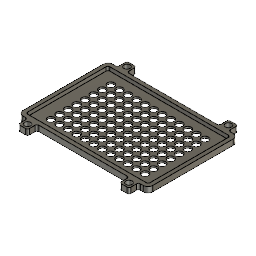
Assembled (Autodesk Fusion 360 archive; units mm, degrees)
design "Plate_Adapter_96"
Autodesk Fusion 360 part; units mm, degrees
note: some values were not read from the file. Chosen so that the rebuilt part matches the saved one: which face or edge a step refers to; which pieces of a blend or face edit are solid. Set by a fixed rule: which sketch regions a step uses.
sketch "Sketch1" plane through (0, 0, 0) normal (0, 0, 1) x (1, 0, 0)
  line L0 (-68.38, 47.37) -> (68.38, 47.37)
  line L1 (68.38, 47.37) -> (68.38, -47.37)
  line L2 (68.38, -47.37) -> (-68.38, -47.37)
  line L3 (-68.38, -47.37) -> (-68.38, 47.37)
  line L4 (-68.38, 47.37) -> (68.38, -47.37) construction
  line L5 (68.38, 47.37) -> (-68.38, -47.37) construction
  line L6 (-58.38, 57.37) -> (-48.38, 57.37)
  line L7 (-48.38, 57.37) -> (-48.38, 47.37)
  line L8 (-48.38, 47.37) -> (-58.38, 47.37)
  line L9 (-58.38, 47.37) -> (-58.38, 57.37)
  line L10 (48.38, 57.37) -> (58.38, 57.37)
  line L11 (58.38, 57.37) -> (58.38, 47.37)
  line L12 (58.38, 47.37) -> (48.38, 47.37)
  line L13 (48.38, 47.37) -> (48.38, 57.37)
  line L14 (48.38, -47.37) -> (58.38, -47.37)
  line L15 (58.38, -47.37) -> (58.38, -57.37)
  line L16 (58.38, -57.37) -> (48.38, -57.37)
  line L17 (48.38, -57.37) -> (48.38, -47.37)
  line L18 (-58.38, -47.37) -> (-48.38, -47.37)
  line L19 (-48.38, -47.37) -> (-48.38, -57.37)
  line L20 (-48.38, -57.37) -> (-58.38, -57.37)
  line L21 (-58.38, -57.37) -> (-58.38, -47.37)
  line L22 (-49.5, 31.5) -> (49.5, 31.5)
  line L23 (49.5, 31.5) -> (49.5, -31.5)
  line L24 (49.5, -31.5) -> (-49.5, -31.5)
  line L25 (-49.5, -31.5) -> (-49.5, 31.5)
  line L26 (-49.5, 31.5) -> (49.5, -31.5) construction
  line L27 (49.5, 31.5) -> (-49.5, -31.5) construction
  circle A0 centre (-49.5, -31.5) radius 3.575
  circle A1 centre (-40.5, -31.5) radius 3.575
  circle A2 centre (-31.5, -31.5) radius 3.575
  circle A3 centre (-22.5, -31.5) radius 3.575
  circle A4 centre (-13.5, -31.5) radius 3.575
  circle A5 centre (-4.5, -31.5) radius 3.575
  circle A6 centre (4.5, -31.5) radius 3.575
  circle A7 centre (13.5, -31.5) radius 3.575
  circle A8 centre (22.5, -31.5) radius 3.575
  circle A9 centre (31.5, -31.5) radius 3.575
  circle A10 centre (40.5, -31.5) radius 3.575
  circle A11 centre (49.5, -31.5) radius 3.575
  circle A12 centre (-49.5, -22.5) radius 3.575
  circle A13 centre (-40.5, -22.5) radius 3.575
  circle A14 centre (-31.5, -22.5) radius 3.575
  circle A15 centre (-22.5, -22.5) radius 3.575
  circle A16 centre (-13.5, -22.5) radius 3.575
  circle A17 centre (-4.5, -22.5) radius 3.575
  circle A18 centre (4.5, -22.5) radius 3.575
  circle A19 centre (13.5, -22.5) radius 3.575
  circle A20 centre (22.5, -22.5) radius 3.575
  circle A21 centre (31.5, -22.5) radius 3.575
  circle A22 centre (40.5, -22.5) radius 3.575
  circle A23 centre (49.5, -22.5) radius 3.575
  circle A24 centre (-49.5, -13.5) radius 3.575
  circle A25 centre (-40.5, -13.5) radius 3.575
  circle A26 centre (-31.5, -13.5) radius 3.575
  circle A27 centre (-22.5, -13.5) radius 3.575
  circle A28 centre (-13.5, -13.5) radius 3.575
  circle A29 centre (-4.5, -13.5) radius 3.575
  circle A30 centre (4.5, -13.5) radius 3.575
  circle A31 centre (13.5, -13.5) radius 3.575
  circle A32 centre (22.5, -13.5) radius 3.575
  circle A33 centre (31.5, -13.5) radius 3.575
  circle A34 centre (40.5, -13.5) radius 3.575
  circle A35 centre (49.5, -13.5) radius 3.575
  circle A36 centre (-49.5, -4.5) radius 3.575
  circle A37 centre (-40.5, -4.5) radius 3.575
  circle A38 centre (-31.5, -4.5) radius 3.575
  circle A39 centre (-22.5, -4.5) radius 3.575
  circle A40 centre (-13.5, -4.5) radius 3.575
  circle A41 centre (-4.5, -4.5) radius 3.575
  circle A42 centre (4.5, -4.5) radius 3.575
  circle A43 centre (13.5, -4.5) radius 3.575
  circle A44 centre (22.5, -4.5) radius 3.575
  circle A45 centre (31.5, -4.5) radius 3.575
  circle A46 centre (40.5, -4.5) radius 3.575
  circle A47 centre (49.5, -4.5) radius 3.575
  circle A48 centre (-49.5, 4.5) radius 3.575
  circle A49 centre (-40.5, 4.5) radius 3.575
  circle A50 centre (-31.5, 4.5) radius 3.575
  circle A51 centre (-22.5, 4.5) radius 3.575
  circle A52 centre (-13.5, 4.5) radius 3.575
  circle A53 centre (-4.5, 4.5) radius 3.575
  circle A54 centre (4.5, 4.5) radius 3.575
  circle A55 centre (13.5, 4.5) radius 3.575
  circle A56 centre (22.5, 4.5) radius 3.575
  circle A57 centre (31.5, 4.5) radius 3.575
  circle A58 centre (40.5, 4.5) radius 3.575
  circle A59 centre (49.5, 4.5) radius 3.575
  circle A60 centre (-49.5, 13.5) radius 3.575
  circle A61 centre (-40.5, 13.5) radius 3.575
  circle A62 centre (-31.5, 13.5) radius 3.575
  circle A63 centre (-22.5, 13.5) radius 3.575
  circle A64 centre (-13.5, 13.5) radius 3.575
  circle A65 centre (-4.5, 13.5) radius 3.575
  circle A66 centre (4.5, 13.5) radius 3.575
  circle A67 centre (13.5, 13.5) radius 3.575
  circle A68 centre (22.5, 13.5) radius 3.575
  circle A69 centre (31.5, 13.5) radius 3.575
  circle A70 centre (40.5, 13.5) radius 3.575
  circle A71 centre (49.5, 13.5) radius 3.575
  circle A72 centre (-49.5, 22.5) radius 3.575
  circle A73 centre (-40.5, 22.5) radius 3.575
  circle A74 centre (-31.5, 22.5) radius 3.575
  circle A75 centre (-22.5, 22.5) radius 3.575
  circle A76 centre (-13.5, 22.5) radius 3.575
  circle A77 centre (-4.5, 22.5) radius 3.575
  circle A78 centre (4.5, 22.5) radius 3.575
  circle A79 centre (13.5, 22.5) radius 3.575
  circle A80 centre (22.5, 22.5) radius 3.575
  circle A81 centre (31.5, 22.5) radius 3.575
  circle A82 centre (40.5, 22.5) radius 3.575
  circle A83 centre (49.5, 22.5) radius 3.575
  circle A84 centre (-49.5, 31.5) radius 3.575
  circle A85 centre (-40.5, 31.5) radius 3.575
  circle A86 centre (-31.5, 31.5) radius 3.575
  circle A87 centre (-22.5, 31.5) radius 3.575
  circle A88 centre (-13.5, 31.5) radius 3.575
  circle A89 centre (-4.5, 31.5) radius 3.575
  circle A90 centre (4.5, 31.5) radius 3.575
  circle A91 centre (13.5, 31.5) radius 3.575
  circle A92 centre (22.5, 31.5) radius 3.575
  circle A93 centre (31.5, 31.5) radius 3.575
  circle A94 centre (40.5, 31.5) radius 3.575
  circle A95 centre (49.5, 31.5) radius 3.575
  point P0 (-57.3369, -42.2056)
  point P1 (-53.88, -84.89)
  dimension "d1" = 136.76
  dimension "d2" = 94.74
  dimension "d3" = 10
  dimension "d4" = 10
  dimension "d5" = 10
  dimension "d6" = 10
  dimension "d7" = 63
  dimension "d8" = 99
  dimension "d10" = 7.15
  dimension "d13" = 99
  dimension "d14" = 63
  constraint perpendicular L0 L1
  constraint parallel L0 L2
  constraint parallel L1 L3
  constraint horizontal L0
  constraint coincident L4 origin
  constraint coincident L5 origin
  constraint horizontal L6
  constraint vertical L7
  constraint horizontal L8
  constraint vertical L9
  constraint coincident L0 L7.end
  constraint horizontal L10
  constraint vertical L11
  constraint horizontal L12
  constraint vertical L13
  constraint horizontal L14
  constraint vertical L15
  constraint horizontal L16
  constraint vertical L17
  constraint horizontal L18
  constraint vertical L19
  constraint horizontal L20
  constraint vertical L21
  constraint perpendicular L22 L23
  constraint parallel L22 L24
  constraint parallel L23 L25
  constraint horizontal L22
  constraint coincident L26 origin
  constraint coincident L27 origin
  measures "d1" distance of L1 L3
  measures "d2" distance of L0.start L2.end
  measures "d3" distance of L6.start L6.end
  measures "d4" distance of L6.start L8.end
  measures "d5" distance of L10.start L10.end
  measures "d6" distance of L10.start L12.end
  measures "d7" distance of L22.end L23.end
  measures "d8" distance of L23.end L24.end
  measures "d10" diameter of A0
extrude "Extrude1" add sketch "Sketch1" along normal mid plane 6 contours L0 L1 L2 L3 L8 L12 L14 L18 | L0 L6 L7 L8 L9 | L2 L18 L19 L20 L21 | L0 L10 L11 L12 L13 | L2 L14 L15 L16 L17 | L22 L23 L24 L25 A0 A1 A2 A3 A4 A5 A6 A7 A8 A9 A10 A11 A12 A23 A24 A35 A36 A47 A48 A59 A60 A71 A72 A83 A84 A85 A86 A87 A88 A89 A90 A91 A92 A93 A94 A95
ref_plane "WorkPlane1" through (0, 0, 3) normal (0, 0, 1) x (1, 0, 0)
sketch "Sketch2" plane through (0, 0, 3) normal (0, 0, 1) x (1, 0, 0)
  line L0 (-64.38, 43.235) -> (64.38, 43.235)
  line L1 (64.38, 43.235) -> (64.38, -43.235)
  line L2 (64.38, -43.235) -> (-64.38, -43.235)
  line L3 (-64.38, -43.235) -> (-64.38, 43.235)
  line L4 (-64.38, 43.235) -> (64.38, -43.235) construction
  line L5 (64.38, 43.235) -> (-64.38, -43.235) construction
  dimension "d18" = 128.76
  dimension "d19" = 86.47
  constraint perpendicular L0 L1
  constraint parallel L0 L2
  constraint parallel L1 L3
  constraint horizontal L0
  constraint coincident L4 origin
  constraint coincident L5 origin
  measures "d18" distance of L1.end L2.end
  measures "d19" distance of L0.end L1.end
extrude "Extrude2" cut sketch "Sketch2" against normal blind 4
sketch "Sketch3" plane through (0, 0, 3) normal (0, 0, 1) x (-1, 0, 0)
  line L0 (-64.38, -43.235) -> (-64.38, 43.235)
  line L1 (-64.38, 43.235) -> (64.38, 43.235)
  line L2 (64.38, 43.235) -> (64.38, -43.235)
  line L3 (64.38, -43.235) -> (-64.38, -43.235)
  line L4 (58.38, 57.37) -> (48.38, 57.37)
  line L5 (48.38, 57.37) -> (48.38, 47.37)
  line L6 (48.38, 47.37) -> (-48.38, 47.37)
  line L7 (-48.38, 47.37) -> (-48.38, 57.37)
  line L8 (-48.38, 57.37) -> (-58.38, 57.37)
  line L9 (-58.38, 57.37) -> (-58.38, 47.37)
  line L10 (-58.38, 47.37) -> (-68.38, 47.37)
  line L11 (-68.38, 47.37) -> (-68.38, -47.37)
  line L12 (-68.38, -47.37) -> (-58.38, -47.37)
  line L13 (-58.38, -47.37) -> (-58.38, -57.37)
  line L14 (-58.38, -57.37) -> (-48.38, -57.37)
  line L15 (-48.38, -57.37) -> (-48.38, -47.37)
  line L16 (-48.38, -47.37) -> (48.38, -47.37)
  line L17 (48.38, -47.37) -> (48.38, -57.37)
  line L18 (48.38, -57.37) -> (58.38, -57.37)
  line L19 (58.38, -57.37) -> (58.38, -47.37)
  line L20 (58.38, -47.37) -> (68.38, -47.37)
  line L21 (68.38, -47.37) -> (68.38, 47.37)
  line L22 (68.38, 47.37) -> (58.38, 47.37)
  line L23 (58.38, 47.37) -> (58.38, 57.37)
  circle A0 centre (53.38, -52.37) radius 3.25
  circle A1 centre (-53.38, -52.3704) radius 3.25
  circle A2 centre (-53.38, 52.3703) radius 3.25
  circle A3 centre (53.38, 52.37) radius 3.25
  dimension "d22" = 6.5
  dimension "d23" = 6.5
  dimension "d24" = 6.5
  dimension "d25" = 6.5
  measures "d22" diameter of A0
  measures "d23" diameter of A1
  measures "d24" diameter of A2
  measures "d25" diameter of A3
extrude "Extrude3" cut sketch "Sketch3" against normal blind 6 contours A0 | A1 | A2 | A3
fillet "Fillet1" radius 5 4 edges at (68.38, -47.37, 0) (68.38, 47.37, 0) (-68.38, -47.37, 0) (-68.38, 47.37, 0)
fillet "Fillet2" radius 2 4 edges at (64.38, 43.235, 1) (-64.38, 43.235, 1) (-64.38, -43.235, 1) (64.38, -43.235, 1)
fillet "Fillet3" radius 2 16 edges at (48.38, 47.37, 0) (48.38, 57.37, 0) (58.38, 57.37, 0) (-58.38, 47.37, 0) (-58.38, 57.37, 0) (-48.38, 57.37, 0) (-48.38, 47.37, 0) (58.38, 47.37, 0) (58.38, -47.37, 0) (58.38, -57.37, 0) (48.38, -57.37, 0) (-48.38, -47.37, 0) (-48.38, -57.37, 0) (48.38, -47.37, 0) (-58.38, -47.37, 0) (-58.38, -57.37, 0)

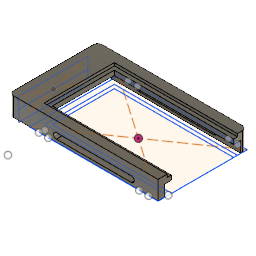
design "Mounting_plate_96_v3 (no bolt holes)"
Autodesk Fusion 360 part; units mm, degrees
sketch "Sketch1" plane through (0, 0, 0) normal (0, 0, 1) x (1, 0, 0)
  line L0 (-68.38, 47.37) -> (68.38, 47.37)
  line L1 (68.38, 47.37) -> (68.38, -47.37)
  line L2 (68.38, -47.37) -> (-68.38, -47.37)
  line L3 (-68.38, -47.37) -> (-68.38, 47.37)
  line L4 (-68.38, 47.37) -> (68.38, -47.37) construction
  line L5 (68.38, 47.37) -> (-68.38, -47.37) construction
  line L6 (-48.38, 47.37) -> (-58.38, 47.37)
  line L7 (58.38, 47.37) -> (48.38, 47.37)
  line L8 (48.38, -47.37) -> (58.38, -47.37)
  line L9 (-58.38, -47.37) -> (-48.38, -47.37)
  line L10 (68.38, 47.37) -> (68.38, 37)
  line L11 (68.38, -47.37) -> (68.38, -36.63)
  line L12 (68.38, 37) -> (-62.58, 37)
  line L13 (-62.58, 37) -> (-62.58, -37)
  line L14 (-62.58, -37) -> (68.38, -37)
  line L15 (68.38, -37) -> (68.38, 37)
  line L16 (68.38, 37) -> (68.38, 33)
  line L17 (68.38, 33) -> (-58.58, 33)
  line L18 (-58.58, 33) -> (-58.58, -33)
  line L19 (-58.58, -33) -> (68.38, -33)
  line L20 (68.38, -33) -> (68.38, 33)
  point P0 (-57.3369, -42.2056)
  point P1 (-53.88, -84.89)
  dimension "d1" = 136.76
  dimension "d2" = 94.74
  dimension "d15" = 10.37
  dimension "d16" = 10.74
  dimension "d17" = 74
  dimension "d18" = 130.96
  dimension "d19" = 4
  dimension "d20" = 66
  dimension "d21" = 126.96
  constraint perpendicular L0 L1
  constraint parallel L0 L2
  constraint parallel L1 L3
  constraint horizontal L0
  constraint horizontal L6
  constraint coincident L0 L6.start
  constraint horizontal L7
  constraint horizontal L8
  constraint horizontal L9
  constraint perpendicular L0 L10
  constraint perpendicular L2 L11
  constraint horizontal L12
  constraint vertical L13
  constraint horizontal L14
  constraint vertical L15
  constraint perpendicular L12 L16
  constraint horizontal L17
  constraint vertical L18
  constraint horizontal L19
  constraint vertical L20
  measures "d1" distance of L1 L3
  measures "d2" distance of L0.start L2.end
  measures "d15" distance of L0.end L10.end
  measures "d16" distance of L1.end L11.end
  measures "d17" distance of L10.end L14.end
  measures "d18" distance of L10.end L12.end
  measures "d19" distance of L10.end L16.end
  measures "d20" distance of L16.end L19.end
  measures "d21" distance of L16.end L17.end
  measures "d160" distance of L0.end
extrude "Extrude2" add sketch "Sketch1" along normal blind 20 contours L0 L1 L2 L3 L6 L7 L8 L9 L10 L11 L12 L13 L14 | L1 L11 L12 L13 L14 L15 L16 L17 L18 L19
ref_plane "WorkPlane2" through (0, 0, 20) normal (0, 0, 1) x (1, 0, 0)
sketch "Sketch4" plane through (0, 0, 20) normal (0, 0, 1) x (1, 0, 0)
  line L0 (68.38, 37) -> (-62.58, 37)
  line L1 (-62.58, 37) -> (-62.58, -37.7)
  line L2 (-62.58, -37.7) -> (68.38, -37.7)
  line L3 (68.38, -37.7) -> (68.38, 37)
  dimension "d30" = 130.96
  dimension "d31" = 74.7
  constraint horizontal L0
  constraint vertical L1
  constraint horizontal L2
  constraint vertical L3
  measures "d30" distance of L0.start L0.end
  measures "d31" distance of L0.start L2.end
extrude "Extrude3" cut sketch "Sketch4" against normal blind 3
ref_plane "WorkPlane3" through (0, 0, 20) normal (0, 0, 1) x (1, 0, 0)
sketch "Sketch5" plane through (0, 0, 20) normal (0, 0, 1) x (1, 0, 0)
  circle A0 centre (-53.38, 52.37) radius 3.25
  circle A1 centre (53.38, 52.37) radius 3.25
  circle A2 centre (-53.38, -52.37) radius 3.25
  circle A3 centre (53.38, -52.37) radius 3.25
  dimension "d35" = 6.5
  dimension "d38" = 106.76
  dimension "d39" = -104.74
  measures "d35" diameter of A0
extrude "Extrude4" cut sketch "Sketch5" against normal blind 20
ref_plane "WorkPlane5" through (68.38, 0, 0) normal (1, 0, 0) x (0, 1, 0)
ref_plane "WorkPlane6" through (68.38, 0, 0) normal (1, 0, 0) x (0, 1, 0)
sketch "Sketch7" plane through (68.38, 0, 0) normal (1, 0, 0) x (0, 1, 0)
  line L0 (40.5, 12) -> (-40.5, 12)
  line L1 (-40.5, 12) -> (-40.5, -12)
  line L2 (-40.5, -12) -> (40.5, -12)
  line L3 (40.5, -12) -> (40.5, 12)
  line L4 (40.5, 12) -> (-40.5, -12) construction
  line L5 (-40.5, 12) -> (40.5, -12) construction
  dimension "d45" = 81
  dimension "d46" = 24
  constraint perpendicular L0 L1
  constraint parallel L0 L2
  constraint parallel L1 L3
  constraint horizontal L0
  constraint coincident L4 origin
  constraint coincident L5 origin
  measures "d45" distance of L1.end L2.end
  measures "d46" distance of L0.end L1.end
extrude "Extrude5" cut sketch "Sketch7" against normal blind 136.76
fillet "Fillet2" [no effect]
ref_plane "WorkPlane7" through (0, -47.37, 10) normal (0, -1, 0) x (1, 0, 0)
delete_face "DeleteFace1" [no effect]
ref_plane "WorkPlane9" through (0, -47.37, 10) normal (0, -1, 0) x (1, 0, 0)
sketch "Sketch10" plane through (0, -47.37, 10) normal (0, -1, 0) x (1, 0, 0)
  line L0 (0, -10) -> (0, -4)
  line L1 (40, -7) -> (-40, -7)
  line L2 (-40, -7) -> (-40, -1)
  line L3 (-40, -1) -> (40, -1)
  line L4 (40, -1) -> (40, -7)
  line L5 (40, -7) -> (-40, -1) construction
  line L6 (-40, -7) -> (40, -1) construction
  circle A0 centre (-40, -4) radius 3
  circle A1 centre (40, -4) radius 3
  point P0 (0, -4)
  dimension "d72" = 6
  dimension "d73" = 6
  dimension "d74" = 80
  dimension "d75" = 6
  dimension "d76" = 6
  constraint vertical L0
  constraint perpendicular L1 L2
  constraint parallel L1 L3
  constraint parallel L2 L4
  constraint horizontal L1
  constraint coincident L5 P0
  constraint coincident L6 P0
  constraint coincident P0 L0.end
  constraint midpoint L2 A0.centre
  constraint midpoint L4 A1.centre
  measures "d72" distance of L0.start P0
  measures "d73" distance of L1.end L2.end
  measures "d74" distance of L2.end L3.end
  measures "d75" diameter of A0
  measures "d76" diameter of A1
extrude "Extrude9" cut sketch "Sketch10" against normal blind 6.87
ref_plane "WorkPlane10" through (0, 47.37, 10) normal (0, 1, 0) x (-1, 0, 0)
sketch "Sketch11" plane through (0, 47.37, 10) normal (0, 1, 0) x (1, 0, 0)
  line L0 (0, 10) -> (0, 4)
  line L1 (-40, 7) -> (40, 7)
  line L2 (40, 7) -> (40, 1)
  line L3 (40, 1) -> (-40, 1)
  line L4 (-40, 1) -> (-40, 7)
  line L5 (-40, 7) -> (40, 1) construction
  line L6 (40, 7) -> (-40, 1) construction
  circle A0 centre (40, 4) radius 3
  circle A1 centre (-40, 4) radius 3
  point P0 (0, 4)
  dimension "d80" = 6
  dimension "d81" = 80
  dimension "d82" = 6
  dimension "d83" = 6
  dimension "d84" = 6
  constraint vertical L0
  constraint perpendicular L1 L2
  constraint parallel L1 L3
  constraint parallel L2 L4
  constraint horizontal L1
  constraint coincident L5 P0
  constraint coincident L6 P0
  constraint coincident P0 L0.end
  constraint midpoint L2 A0.centre
  constraint midpoint L4 A1.centre
  measures "d80" distance of L0.start P0
  measures "d81" distance of L2.end L3.end
  measures "d82" distance of L1.end L2.end
  measures "d83" diameter of A0
  measures "d84" diameter of A1
extrude "Extrude10" cut sketch "Sketch11" against normal blind 6.87
ref_plane "WorkPlane11" through (0, 0, 0) normal (0, 0, 1) x (1, 0, 0)
sketch "Sketch12" plane through (0, 0, 0) normal (0, 0, 1) x (1, 0, 0)
ref_plane "WorkPlane12" through (-68.38, 0, 10) normal (-1, 0, 0) x (0, -1, 0)
ref_plane "WorkPlane13" through (-68.38, 0, 10) normal (-1, 0, 0) x (0, -1, 0)
sketch "Sketch19" plane through (68.38, 0, 0) normal (1, 0, 0) x (0, 1, 0)
ref_plane "WorkPlane19" through (-68.38, 0, 10) normal (-1, 0, 0) x (0, -1, 0)
sketch "Sketch21" plane through (-68.38, 0, 10) normal (-1, 0, 0) x (0, 1, 0)
  line L0 (42, -2) -> (-42, -2)
  line L1 (42, -2) -> (-42, 22) construction
  line L2 (-42, -2) -> (42, 22) construction
  line L3 (42, -2) -> (-42, -2)
  line L4 (-42, -2) -> (-42, 10)
  line L5 (-42, 10) -> (42, 10)
  line L6 (42, 10) -> (42, -2)
  point P0 (0, 10)
  dimension "d112" = 84
  dimension "d113" = 24
  constraint horizontal L0
  constraint coincident L1 P0
  constraint coincident L2 P0
  constraint horizontal L3
  constraint vertical L4
  constraint horizontal L5
  constraint vertical L6
  measures "d112" distance of L1.end L2.end
  measures "d113" distance of L0.end L1.end
ref_plane "WorkPlane25" through (-68.38, 0, 10) normal (-1, 0, 0) x (0, -1, 0)
sketch "Sketch27" plane through (-68.38, 0, 10) normal (-1, 0, 0) x (0, 1, 0)
  line L0 (-47.37, 30) -> (47.37, 30)
  line L1 (47.37, 30) -> (47.37, -10)
  line L2 (47.37, -10) -> (-47.37, -10)
  line L3 (-47.37, -10) -> (-47.37, 30)
  line L4 (-47.37, 30) -> (47.37, -10) construction
  line L5 (47.37, 30) -> (-47.37, -10) construction
  line L6 (47.37, 10) -> (-47.37, 10)
  point P0 (0, 10)
  dimension "d149" = 94.74
  dimension "d150" = 40
  constraint perpendicular L0 L1
  constraint parallel L0 L2
  constraint parallel L1 L3
  constraint horizontal L0
  constraint coincident L4 P0
  constraint coincident L5 P0
  constraint midpoint L1 L6.start
  constraint midpoint L3 L6.end
  measures "d149" distance of L1.end L2.end
  measures "d150" distance of L0.end L1.end
extrude "Extrude22" add sketch "Sketch27" along normal blind 22.07 contours L1 L2 L3 L6
ref_plane "WorkPlane26" through (-90.45, 0, 10) normal (-1, 0, 0) x (0, 0, 1)
sketch "Sketch28" plane through (-90.45, 0, 10) normal (-1, 0, 0) x (0, 1, 0)
  line L0 (-36.75, 22) -> (36.75, 22)
  line L1 (36.75, 22) -> (36.75, -2)
  line L2 (36.75, -2) -> (-36.75, -2)
  line L3 (-36.75, -2) -> (-36.75, 22)
  line L4 (-36.75, 22) -> (36.75, -2) construction
  line L5 (36.75, 22) -> (-36.75, -2) construction
  line L6 (36.75, 10) -> (-36.75, 10)
  point P0 (0, 10)
  dimension "d164" = 73.5
  dimension "d165" = 24
  constraint perpendicular L0 L1
  constraint parallel L0 L2
  constraint parallel L1 L3
  constraint horizontal L0
  constraint coincident L4 P0
  constraint coincident L5 P0
  constraint midpoint L1 L6.start
  constraint midpoint L3 L6.end
  measures "d164" distance of L1.end L2.end
  measures "d165" distance of L0.end L1.end
extrude "Extrude25" cut sketch "Sketch28" against normal blind 22.07 contours L1 L2 L3 L6
ref_plane "WorkPlane31" through (-68.38, 0, 10) normal (-1, 0, 0) x (0, 0, 1)
sketch "Sketch33" plane through (-68.38, 0, 10) normal (-1, 0, 0) x (0, 1, 0)
  line L0 (40.5, 22) -> (-40.5, 22)
  line L1 (-40.5, 22) -> (-40.5, -2)
  line L2 (-40.5, -2) -> (40.5, -2)
  line L3 (40.5, -2) -> (40.5, 22)
  line L4 (40.5, 22) -> (-40.5, -2) construction
  line L5 (-40.5, 22) -> (40.5, -2) construction
  point P0 (0, 10)
  dimension "d173" = 81
  dimension "d174" = 24
  constraint perpendicular L0 L1
  constraint parallel L0 L2
  constraint parallel L1 L3
  constraint horizontal L0
  constraint coincident L4 P0
  constraint coincident L5 P0
  measures "d173" distance of L1.end L2.end
  measures "d174" distance of L0.end L1.end
extrude "Extrude26" cut sketch "Sketch33" along normal blind 15.2
ref_plane "WorkPlane32" through (-11.035, 0, 12) normal (0, 0, -1) x (0, -1, 0)
fillet "Fillet6" radius 5 3 edges at (-90.45, 47.37, 10) (-90.45, -47.37, 10) (68.38, 47.37, 10)
sketch "Sketch34" plane through (-11.035, 0, 12) normal (0, 0, -1) x (1, 0, 0)
  line L0 (-72.545, -36.75) -> (-86.285, -36.75)
  line L1 (-86.285, -36.75) -> (-86.285, 36.75)
  line L2 (-86.285, 36.75) -> (-72.545, 36.75)
  line L3 (-72.545, 36.75) -> (-72.545, -36.75)
  line L4 (-72.545, -36.75) -> (-86.285, 36.75) construction
  line L5 (-86.285, -36.75) -> (-72.545, 36.75) construction
  point P0 (-79.415, 0)
  dimension "d178" = 13.74
  dimension "d179" = 73.5
  constraint perpendicular L0 L1
  constraint parallel L0 L2
  constraint parallel L1 L3
  constraint horizontal L0
  constraint coincident L4 P0
  constraint coincident L5 P0
  measures "d178" distance of L1.end L2.end
  measures "d179" distance of L0.end L1.end
extrude "Extrude27" [suppressed]
ref_plane "WorkPlane27" through (-68.38, 0, 0) normal (1, 0, 0) x (0, 1, 0)
sketch "Sketch29" plane through (-68.38, 0, 0) normal (1, 0, 0) x (0, 1, 0)
  line L0 (40.5, 12) -> (-40.5, 12)
  line L1 (-40.5, 12) -> (-40.5, -12)
  line L2 (-40.5, -12) -> (40.5, -12)
  line L3 (40.5, -12) -> (40.5, 12)
  line L4 (40.5, 12) -> (-40.5, -12) construction
  line L5 (-40.5, 12) -> (40.5, -12) construction
  dimension "d159" = 24
  dimension "d160" = 81
  constraint perpendicular L0 L1
  constraint parallel L0 L2
  constraint parallel L1 L3
  constraint horizontal L0
  constraint coincident L4 origin
  constraint coincident L5 origin
  measures "d159" distance of L0.end L1.end
  measures "d160" distance of L1.end L2.end
extrude "Extrude24" [suppressed]
ref_plane "WorkPlane28" through (-11.035, 0, 12) normal (0, 0, -1) x (0, -1, 0)
sketch "Sketch30" plane through (-11.035, 0, 12) normal (0, 0, -1) x (1, 0, 0)
extrude "Extrude15" [suppressed]
ref_plane "WorkPlane20" through (-68.32, 0, 0) normal (1, 0, 0) x (0, 1, 0)
sketch "Sketch22" plane through (-68.32, 0, 0) normal (1, 0, 0) x (0, 1, 0)
  line L0 (40.5, -12) -> (-40.5, -12)
  line L1 (-40.5, -12) -> (-40.5, 12)
  line L2 (-40.5, 12) -> (40.5, 12)
  line L3 (40.5, 12) -> (40.5, -12)
  line L4 (40.5, -12) -> (-40.5, 12) construction
  line L5 (-40.5, -12) -> (40.5, 12) construction
  dimension "d117" = 81
  dimension "d118" = 24
  constraint perpendicular L0 L1
  constraint parallel L0 L2
  constraint parallel L1 L3
  constraint horizontal L0
  constraint coincident L4 origin
  constraint coincident L5 origin
  measures "d117" distance of L1.end L2.end
  measures "d118" distance of L0.end L1.end
extrude "Extrude16" [suppressed]
ref_plane "WorkPlane23" through (-76.98, 0, 12) normal (0, 0, 1) x (0, 1, 0)
sketch "Sketch25" plane through (-76.98, 0, 12) normal (0, 0, 1) x (1, 0, 0)
  line L0 (8.6, 42) -> (-8.6, 42)
  line L1 (-8.6, 42) -> (-8.6, -42)
  line L2 (-8.6, -42) -> (8.6, -42)
  line L3 (8.6, -42) -> (8.6, 42)
  dimension "d136" = 17.2
  dimension "d137" = 84
  constraint horizontal L0
  constraint vertical L1
  constraint horizontal L2
  constraint vertical L3
  measures "d136" distance of L0.start L0.end
  measures "d137" distance of L0.start L2.end
extrude "Extrude19" [suppressed]
fillet "Fillet5" [suppressed]
ref_plane "WorkPlane24" through (-85.58, 0, 6.5) normal (-1, 0, 0) x (0, -1, 0)
sketch "Sketch26" plane through (-85.58, 0, 6.5) normal (-1, 0, 0) x (0, 1, 0)
  line L0 (38, 18.5) -> (-38, 18.5)
  line L1 (-38, 18.5) -> (-38, -3.5)
  line L2 (-38, -3.5) -> (38, -3.5)
  line L3 (38, -3.5) -> (38, 18.5)
  line L4 (38, 18.5) -> (-38, -3.5) construction
  line L5 (-38, 18.5) -> (38, -3.5) construction
  point P0 (0, 7.5)
  dimension "d142" = 76
  dimension "d143" = 22
  constraint perpendicular L0 L1
  constraint parallel L0 L2
  constraint parallel L1 L3
  constraint horizontal L0
  constraint coincident L4 P0
  constraint coincident L5 P0
  measures "d142" distance of L1.end L2.end
  measures "d143" distance of L0.end L1.end
extrude "Extrude21" [suppressed]
extrude "Extrude20" [suppressed]
fillet "Fillet3" [suppressed]
fillet "Fillet4" [suppressed]
ref_plane "WorkPlane21" through (-85.58, 0, 5) normal (-1, 0, 0) x (0, 0, 1)
ref_plane "WorkPlane22" through (-85.58, 0, 5) normal (-1, 0, 0) x (0, 0, 1)
sketch "Sketch24" plane through (-85.58, 0, 5) normal (-1, 0, 0) x (0, 1, 0)
  line L0 (-38, 11) -> (38, 11)
  line L1 (38, 11) -> (38, -3)
  line L2 (38, -3) -> (-38, -3)
  line L3 (-38, -3) -> (-38, 11)
  line L4 (-38, 11) -> (38, -3) construction
  line L5 (38, 11) -> (-38, -3) construction
  point P0 (0, 4)
  dimension "d131" = 76
  dimension "d132" = 14
  constraint perpendicular L0 L1
  constraint parallel L0 L2
  constraint parallel L1 L3
  constraint horizontal L0
  constraint coincident L4 P0
  constraint coincident L5 P0
  measures "d131" distance of L1.end L2.end
  measures "d132" distance of L0.end L1.end
extrude "Extrude18" [suppressed]

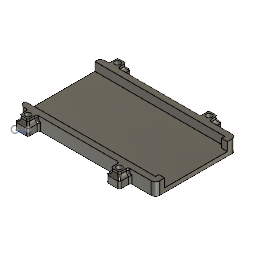
design "Base_96"
Autodesk Fusion 360 part; units mm, degrees
sketch "Sketch1" plane through (0, 0, 0) normal (0, 0, 1) x (1, 0, 0)
  line L0 (-68.38, 47.37) -> (68.38, 47.37)
  line L1 (68.38, 47.37) -> (68.38, -47.37)
  line L2 (68.38, -47.37) -> (-68.38, -47.37)
  line L3 (-68.38, -47.37) -> (-68.38, 47.37)
  line L4 (-68.38, 47.37) -> (68.38, -47.37) construction
  line L5 (68.38, 47.37) -> (-68.38, -47.37) construction
  line L6 (-58.38, 57.37) -> (-48.38, 57.37)
  line L7 (-48.38, 57.37) -> (-48.38, 47.37)
  line L8 (-48.38, 47.37) -> (-58.38, 47.37)
  line L9 (-58.38, 47.37) -> (-58.38, 57.37)
  line L10 (48.38, 57.37) -> (58.38, 57.37)
  line L11 (58.38, 57.37) -> (58.38, 47.37)
  line L12 (58.38, 47.37) -> (48.38, 47.37)
  line L13 (48.38, 47.37) -> (48.38, 57.37)
  line L14 (48.38, -47.37) -> (58.38, -47.37)
  line L15 (58.38, -47.37) -> (58.38, -57.37)
  line L16 (58.38, -57.37) -> (48.38, -57.37)
  line L17 (48.38, -57.37) -> (48.38, -47.37)
  line L18 (-58.38, -47.37) -> (-48.38, -47.37)
  line L19 (-48.38, -47.37) -> (-48.38, -57.37)
  line L20 (-48.38, -57.37) -> (-58.38, -57.37)
  line L21 (-58.38, -57.37) -> (-58.38, -47.37)
  point P0 (-57.3369, -42.2056)
  point P1 (-53.88, -84.89)
  dimension "d1" = 136.76
  dimension "d2" = 94.74
  dimension "d3" = 10
  dimension "d4" = 10
  dimension "d5" = 10
  dimension "d6" = 10
  constraint perpendicular L0 L1
  constraint parallel L0 L2
  constraint parallel L1 L3
  constraint horizontal L0
  constraint horizontal L6
  constraint vertical L7
  constraint horizontal L8
  constraint vertical L9
  constraint coincident L0 L7.end
  constraint horizontal L10
  constraint vertical L11
  constraint horizontal L12
  constraint vertical L13
  constraint horizontal L14
  constraint vertical L15
  constraint horizontal L16
  constraint vertical L17
  constraint horizontal L18
  constraint vertical L19
  constraint horizontal L20
  constraint vertical L21
  measures "d1" distance of L1 L3
  measures "d2" distance of L0.start L2.end
  measures "d3" distance of L6.start L6.end
  measures "d4" distance of L6.start L8.end
  measures "d5" distance of L10.start L10.end
  measures "d6" distance of L10.start L12.end
  measures "d79" distance of L0.end
extrude "Extrude1" add sketch "Sketch1" along normal blind 15
ref_plane "WorkPlane1" through (0, 0, 15) normal (0, 0, 1) x (1, 0, 0)
sketch "Sketch2" plane through (0, 0, 15) normal (0, 0, 1) x (1, 0, 0)
  line L0 (68.38, -40.5) -> (-68.38, -40.5)
  line L1 (-68.38, -40.5) -> (-68.38, 40.5)
  line L2 (-68.38, 40.5) -> (68.38, 40.5)
  line L3 (68.38, 40.5) -> (68.38, -40.5)
  line L4 (68.38, -40.5) -> (-68.38, 40.5) construction
  line L5 (-68.38, -40.5) -> (68.38, 40.5) construction
  dimension "d18" = 136.76
  dimension "d19" = 81
  constraint perpendicular L0 L1
  constraint parallel L0 L2
  constraint parallel L1 L3
  constraint horizontal L0
  constraint coincident L4 origin
  constraint coincident L5 origin
  measures "d18" distance of L1.end L2.end
  measures "d19" distance of L0.end L1.end
extrude "Extrude2" cut sketch "Sketch2" against normal blind 10
ref_plane "WorkPlane2" through (68.38, 0, 7.5) normal (1, 0, 0) x (0, 1, 0)
sketch "Sketch3" plane through (68.38, 0, 7.5) normal (1, 0, 0) x (0, 1, 0)
  line L0 (42, -7.5) -> (-42, -7.5)
  line L1 (-42, -7.5) -> (-42, 7.5)
  line L2 (-42, 7.5) -> (42, 7.5)
  line L3 (42, 7.5) -> (42, -7.5)
  line L4 (42, -7.5) -> (-42, 7.5) construction
  line L5 (-42, -7.5) -> (42, 7.5) construction
  dimension "d23" = 84
  dimension "d24" = 15
  constraint perpendicular L0 L1
  constraint parallel L0 L2
  constraint parallel L1 L3
  constraint horizontal L0
  constraint coincident L4 origin
  constraint coincident L5 origin
  measures "d23" distance of L1.end L2.end
  measures "d24" distance of L0.end L1.end
sketch "Sketch5" plane through (7.88, 0, 15) normal (0, 0, 1) x (1, 0, 0)
  circle A0 centre (-61.26, 52.37) radius 3.25
  circle A1 centre (45.5, 52.37) radius 3.25
  circle A2 centre (-61.26, -52.37) radius 3.25
  circle A3 centre (45.5, -52.37) radius 3.25
  dimension "d29" = 6.5
  dimension "d32" = 106.76
  dimension "d33" = -104.74
  measures "d29" diameter of A0
extrude "Extrude4" cut sketch "Sketch5" against normal blind 15
ref_plane "WorkPlane7" through (68.38, 0, 7.5) normal (1, 0, 0) x (0, 1, 0)
sketch "Sketch8" plane through (68.38, 0, 7.5) normal (1, 0, 0) x (0, 1, 0)
  line L0 (0, -7.5) -> (-42, -7.5)
  line L1 (-42, -7.5) -> (42, -7.5)
  line L2 (42, -7.5) -> (42, 7.5)
  line L3 (42, 7.5) -> (-42, 7.5)
  line L4 (-42, 7.5) -> (-42, -7.5)
  dimension "d52" = 42
  dimension "d53" = 84
  dimension "d54" = 15
  constraint horizontal L0
  constraint horizontal L1
  constraint vertical L2
  constraint horizontal L3
  constraint vertical L4
  measures "d52" distance of L0.start L0.end
  measures "d53" distance of L0.end L1.end
  measures "d54" distance of L0.end L3.end
ref_plane "WorkPlane12" through (68.38, 0, 7.5) normal (1, 0, 0) x (0, 1, 0)
sketch "Sketch13" plane through (68.38, 0, 7.5) normal (1, 0, 0) x (0, 1, 0)
  line L0 (47.37, -22.5) -> (-47.37, -22.5)
  line L1 (-47.37, -22.5) -> (-47.37, 7.5)
  line L2 (-47.37, 7.5) -> (47.37, 7.5)
  line L3 (47.37, 7.5) -> (47.37, -22.5)
  line L4 (47.37, -22.5) -> (-47.37, 7.5) construction
  line L5 (-47.37, -22.5) -> (47.37, 7.5) construction
  line L6 (-47.37, -7.5) -> (47.37, -7.5)
  point P0 (0, -7.5)
  dimension "d78" = 94.74
  dimension "d79" = 30
  constraint perpendicular L0 L1
  constraint parallel L0 L2
  constraint parallel L1 L3
  constraint horizontal L0
  constraint coincident L4 P0
  constraint coincident L5 P0
  constraint midpoint L1 L6.start
  constraint midpoint L3 L6.end
  measures "d78" distance of L1.end L2.end
  measures "d79" distance of L0.end L1.end
extrude "Extrude10" add sketch "Sketch13" along normal blind 22.07 contours L1 L2 L3 L6
ref_plane "WorkPlane13" through (90.45, 0, 7.5) normal (1, 0, 0) x (0, 0, -1)
ref_plane "WorkPlane15" through (68.38, 0, 10) normal (-1, 0, 0) x (0, -1, 0)
sketch "Sketch17" plane through (68.38, 0, 0) normal (-1, 0, 0) x (0, -1, 0)
  line L0 (40.5, 5) -> (40.5, 15)
  line L1 (40.5, 15) -> (-40.5, 15)
  line L2 (-40.5, 15) -> (-40.5, 5)
  line L3 (-40.5, 5) -> (40.5, 5)
  line L4 (40.5, 5) -> (-40.5, 5)
  line L5 (-40.5, 5) -> (-40.5, 25)
  line L6 (-40.5, 25) -> (40.5, 25)
  line L7 (40.5, 25) -> (40.5, 5)
  line L8 (40.5, 5) -> (-40.5, 25) construction
  line L9 (-40.5, 5) -> (40.5, 25) construction
  point P0 (0, 15)
  dimension "d93" = 81
  dimension "d94" = 20
  constraint perpendicular L4 L5
  constraint parallel L4 L6
  constraint parallel L5 L7
  constraint horizontal L4
  constraint coincident L8 P0
  constraint coincident L9 P0
  constraint midpoint L1 P0
  measures "d93" distance of L5.end L6.end
  measures "d94" distance of L2.end L5.end
extrude "Extrude13" cut sketch "Sketch17" against normal blind 15.2 contours L0 L1 L2 L3 L4 L5 L7
sketch "Sketch14" plane through (90.45, 0, 7.5) normal (1, 0, 0) x (0, 1, 0)
  line L0 (36.75, -2.5) -> (-36.75, -2.5)
  line L1 (-36.75, -2.5) -> (-36.75, 17.5)
  line L2 (-36.75, 17.5) -> (36.75, 17.5)
  line L3 (36.75, 17.5) -> (36.75, -2.5)
  line L4 (36.75, -2.5) -> (-36.75, 17.5) construction
  line L5 (-36.75, -2.5) -> (36.75, 17.5) construction
  line L6 (-36.75, 7.5) -> (36.75, 7.5)
  point P0 (0, 7.5)
  dimension "d83" = 73.5
  dimension "d84" = 20
  constraint perpendicular L0 L1
  constraint parallel L0 L2
  constraint parallel L1 L3
  constraint horizontal L0
  constraint coincident L4 P0
  constraint coincident L5 P0
  constraint midpoint L1 L6.start
  constraint midpoint L3 L6.end
  measures "d83" distance of L1.end L2.end
  measures "d84" distance of L0.end L1.end
extrude "Extrude11" cut sketch "Sketch14" against normal blind 32.07 contours L0 L1 L3 L6
fillet "Fillet9" radius 5 4 edges at (-68.38, -47.37, 7.5) (90.45, -47.37, 7.5) (90.45, 47.37, 7.5) (-68.38, 47.37, 7.5)
ref_plane "WorkPlane16" through (0, 0, 0) normal (0, 0, 1) x (1, 0, 0)
sketch "Sketch18" plane through (0, 0, 0) normal (0, 0, 1) x (1, 0, 0)
  line L0 (-58.38, -57.37) -> (-53.38, -57.37)
  line L1 (-53.38, -57.37) -> (-53.38, -52.37)
  line L2 (-45.63, -60.12) -> (-61.13, -60.12)
  line L3 (-61.13, -60.12) -> (-61.13, -44.62)
  line L4 (-61.13, -44.62) -> (-45.63, -44.62)
  line L5 (-45.63, -44.62) -> (-45.63, -60.12)
  line L6 (-45.63, -60.12) -> (-61.13, -44.62) construction
  line L7 (-61.13, -60.12) -> (-45.63, -44.62) construction
  line L8 (45.63, -44.62) -> (61.13, -44.62)
  line L9 (45.63, -60.12) -> (45.63, -44.62)
  line L10 (61.13, -60.12) -> (45.63, -60.12)
  line L11 (61.13, -44.62) -> (61.13, -60.12)
  line L12 (-61.13, 60.12) -> (-45.63, 60.12)
  line L13 (-61.13, 44.62) -> (-61.13, 60.12)
  line L14 (-45.63, 44.62) -> (-61.13, 44.62)
  line L15 (-45.63, 60.12) -> (-45.63, 44.62)
  line L16 (45.63, 60.12) -> (61.13, 60.12)
  line L17 (45.63, 44.62) -> (45.63, 60.12)
  line L18 (61.13, 44.62) -> (45.63, 44.62)
  line L19 (61.13, 60.12) -> (61.13, 44.62)
  point P0 (-53.38, -52.37)
  dimension "d99" = 5
  dimension "d100" = 5
  dimension "d101" = 15.5
  dimension "d102" = 15.5
  dimension "d105" = 106.76
  dimension "d106" = 104.74
  constraint horizontal L0
  constraint perpendicular L0 L1
  constraint perpendicular L2 L3
  constraint parallel L2 L4
  constraint parallel L3 L5
  constraint horizontal L2
  constraint coincident L6 P0
  constraint coincident L7 P0
  constraint coincident P0 L1.end
  measures "d99" distance of L0.start L0.end
  measures "d100" distance of L0.end P0
  measures "d101" distance of L3.end L4.end
  measures "d102" distance of L2.end L3.end
extrude "Extrude14" add sketch "Sketch18" along normal blind 8
fillet "Fillet10" radius 5 12 edges at (48.38, -52.37, 8) (53.38, -57.37, 8) (58.38, -52.37, 8) (-48.38, -52.37, 8) (-53.38, -57.37, 8) (-58.38, -52.37, 8) (-58.38, 52.37, 8) (-53.38, 57.37, 8) (48.38, 52.37, 8) (53.38, 57.37, 8) (-48.38, 52.37, 8) (58.38, 52.37, 8)
extrude "Extrude15" cut 4 faces at (-55.2454, -51.4717, 8) (-55.2454, 53.2683, 8) (51.5146, 53.2683, 8) (51.5146, -51.4717, 8) along direction (0, 0, -1) blind 8
ref_plane "WorkPlane17" through (0, 0, 0) normal (0, 0, 1) x (1, 0, 0)
sketch "Sketch19" plane through (0, 0, 0) normal (0, 0, 1) x (1, 0, 0)
  line L0 (-61, -60) -> (-53.4, -60)
  line L1 (-53.4, -60) -> (-53.4, -52.4)
  dimension "d120" = 7.6
  dimension "d121" = 7.6
  constraint horizontal L0
  constraint perpendicular L0 L1
  measures "d120" distance of L0.start L0.end
  measures "d121" distance of L0.end L1.end
ref_plane "WorkPlane18" through (0, 0, 0) normal (0, 0, 1) x (1, 0, 0)
sketch "Sketch20" plane through (0, 0, 0) normal (0, 0, 1) x (1, 0, 0)
  line L0 (61.13, 60.12) -> (53.38, 60.12)
  line L1 (53.38, 60.12) -> (53.38, 52.37)
  line L2 (47.9798, 49.2235) -> (53.4049, 46.1201)
  line L3 (53.4049, 46.1201) -> (58.805, 49.2666)
  line L4 (58.805, 49.2666) -> (58.7802, 55.5165)
  line L5 (58.7802, 55.5165) -> (53.3551, 58.62)
  line L6 (53.3551, 58.62) -> (47.955, 55.4734)
  line L7 (47.955, 55.4734) -> (47.9798, 49.2235)
  line L8 (-58.805, 55.4734) -> (-58.7802, 49.2235)
  line L9 (-58.7802, 49.2235) -> (-53.3551, 46.1201)
  line L10 (-53.4049, 58.62) -> (-58.805, 55.4734)
  line L11 (-47.9798, 55.5165) -> (-53.4049, 58.62)
  line L12 (-53.3551, 46.1201) -> (-47.955, 49.2666)
  line L13 (-47.955, 49.2666) -> (-47.9798, 55.5165)
  line L14 (47.955, -49.2666) -> (47.9798, -55.5165)
  line L15 (47.9798, -55.5165) -> (53.4049, -58.6199)
  line L16 (53.3551, -46.12) -> (47.955, -49.2666)
  line L17 (58.7802, -49.2235) -> (53.3551, -46.12)
  line L18 (53.4049, -58.6199) -> (58.805, -55.4734)
  line L19 (58.805, -55.4734) -> (58.7802, -49.2235)
  line L20 (-58.805, -49.2666) -> (-58.7802, -55.5165)
  line L21 (-58.7802, -55.5165) -> (-53.3551, -58.6199)
  line L22 (-53.4049, -46.12) -> (-58.805, -49.2666)
  line L23 (-47.9798, -49.2235) -> (-53.4049, -46.12)
  line L24 (-53.3551, -58.6199) -> (-47.955, -55.4734)
  line L25 (-47.955, -55.4734) -> (-47.9798, -49.2235)
  point P0 (53.38, 52.37)
  point P1 (-53.38, 52.37)
  point P2 (-53.38, 52.37)
  point P3 (53.38, -52.37)
  point P4 (53.38, -52.37)
  point P5 (-53.38, -52.37)
  point P6 (-53.38, -52.37)
  dimension "d123" = 7.75
  dimension "d124" = 7.75
  dimension "d125" = 6.25
  dimension "d128" = -106.76
  dimension "d129" = -104.74
  constraint horizontal L0
  constraint perpendicular L0 L1
  constraint coincident P0 L1.end
  measures "d123" distance of L0.start L0.end
  measures "d124" distance of L0.end P0
  measures "d125" distance of L2.start P0
extrude "Extrude16" cut sketch "Sketch20" along normal blind 4
fillet "Fillet11" radius 2 16 edges at (61.13, -47.37, 4) (61.13, -60.12, 4) (45.63, -60.12, 4) (45.63, -47.37, 4) (-45.63, -47.37, 4) (-45.63, -60.12, 4) (-61.13, -47.37, 4) (-61.13, -60.12, 4) (61.13, 47.37, 4) (61.13, 60.12, 4) (45.63, 60.12, 4) (45.63, 47.37, 4) (-61.13, 47.37, 4) (-61.13, 60.12, 4) (-45.63, 60.12, 4) (-45.63, 47.37, 4)
fillet "Fillet13" radius 2 32 edges at (59.0186, 58.0086, 10.0201) (58.38, 57.37, 13.7326) (47.7414, 58.0086, 10.0201) (48.38, 57.37, 13.7326) (47.0028, 47.37, 9.0191) (48.38, 47.37, 13.7326) (-47.7414, 58.0086, 10.0201) (-48.38, 57.37, 13.7326) (-59.0186, 58.0086, 10.0201) (-58.38, 57.37, 13.7326) (-59.7572, 47.37, 9.0191) (-58.38, 47.37, 13.7326) (-59.7572, -47.37, 9.0191) (-58.38, -47.37, 13.7326) (-59.0186, -58.0086, 10.0201) (-58.38, -57.37, 13.7326) (-47.7414, -58.0086, 10.0201) (-48.38, -57.37, 13.7326) (47.0028, -47.37, 9.0191) (48.38, -47.37, 13.7326) (47.7414, -58.0086, 10.0201) (48.38, -57.37, 13.7326) (59.0186, -58.0086, 10.0201) (58.38, -57.37, 13.7326) (-47.0028, -47.37, 9.0191) (-48.38, -47.37, 13.7326) (59.7572, -47.37, 9.0191) (58.38, -47.37, 13.7326) (59.7572, 47.37, 9.0191) (58.38, 47.37, 13.7326) (-47.0028, 47.37, 9.0191) (-48.38, 47.37, 13.7326)

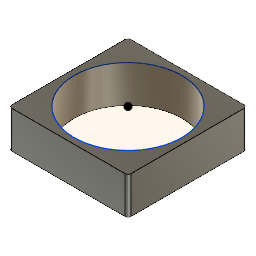
design "Fan"
Autodesk Fusion 360 part; units mm, degrees
sketch "Sketch1" plane through (0, 0, 0) normal (0, 0, 1) x (1, 0, 0)
  line L0 (40, -40) -> (-40, -40)
  line L1 (-40, -40) -> (-40, 40)
  line L2 (-40, 40) -> (40, 40)
  line L3 (40, 40) -> (40, -40)
  line L4 (40, -40) -> (-40, 40) construction
  line L5 (-40, -40) -> (40, 40) construction
  dimension "d1" = 80
  dimension "d2" = 80
  constraint perpendicular L0 L1
  constraint parallel L0 L2
  constraint parallel L1 L3
  constraint horizontal L0
  constraint coincident L4 origin
  constraint coincident L5 origin
  measures "d1" distance of L1.end L2.end
  measures "d2" distance of L0.end L1.end
extrude "Extrude1" add sketch "Sketch1" along normal blind 25
ref_plane "WorkPlane1" through (0, 0, 25) normal (0, 0, 1) x (1, 0, 0)
sketch "Sketch2" plane through (0, 0, 25) normal (0, 0, 1) x (1, 0, 0)
  circle A0 centre (0, 0) radius 36.0555
  constraint coincident A0.centre origin
extrude "Extrude3" cut sketch "Sketch2" against normal blind 25
fillet "Fillet1" radius 2 4 edges at (40, -40, 12.5) (40, 40, 12.5) (-40, 40, 12.5) (-40, -40, 12.5)

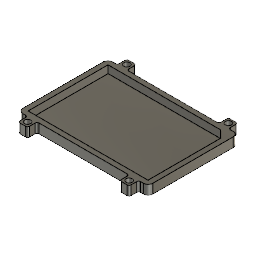
design "Plate_Lid_96"
Autodesk Fusion 360 part; units mm, degrees
sketch "Sketch1" plane through (0, 0, 0) normal (0, 0, 1) x (1, 0, 0)
  line L0 (68.38, -47.235) -> (-68.38, -47.235)
  line L1 (-68.38, -47.235) -> (-68.38, 47.235)
  line L2 (-68.38, 47.235) -> (68.38, 47.235)
  line L3 (68.38, 47.235) -> (68.38, -47.235)
  line L4 (68.38, -47.235) -> (-68.38, 47.235) construction
  line L5 (-68.38, -47.235) -> (68.38, 47.235) construction
  line L6 (-48.38, 47.235) -> (-58.38, 47.235)
  line L7 (-58.38, 47.235) -> (-58.38, 57.235)
  line L8 (-58.38, 57.235) -> (-48.38, 57.235)
  line L9 (-48.38, 57.235) -> (-48.38, 47.235)
  line L10 (-48.38, 47.235) -> (-58.38, 57.235) construction
  line L11 (-58.38, 47.235) -> (-48.38, 57.235) construction
  line L12 (48.38, 57.235) -> (58.38, 57.235)
  line L13 (48.38, 47.235) -> (48.38, 57.235)
  line L14 (58.38, 57.235) -> (58.38, 47.235)
  line L15 (58.38, 47.235) -> (48.38, 47.235)
  line L16 (48.38, -57.235) -> (48.38, -47.235)
  line L17 (48.38, -47.235) -> (58.38, -47.235)
  line L18 (58.38, -47.235) -> (58.38, -57.235)
  line L19 (48.38, -57.235) -> (58.38, -57.235)
  line L20 (-58.38, -57.235) -> (-58.38, -47.235)
  line L21 (-58.38, -47.235) -> (-48.38, -47.235)
  line L22 (-48.38, -47.235) -> (-48.38, -57.235)
  line L23 (-48.38, -57.235) -> (-58.38, -57.235)
  point P0 (-53.38, 52.235)
  dimension "d1" = 136.76
  dimension "d2" = 94.47
  dimension "d3" = 10
  dimension "d4" = 10
  dimension "d6" = 10
  dimension "d7" = 10
  constraint perpendicular L0 L1
  constraint parallel L0 L2
  constraint parallel L1 L3
  constraint horizontal L0
  constraint coincident L4 origin
  constraint coincident L5 origin
  constraint perpendicular L6 L7
  constraint parallel L6 L8
  constraint parallel L7 L9
  constraint horizontal L6
  constraint coincident L10 P0
  constraint coincident L11 P0
  constraint perpendicular L13 L15
  constraint parallel L12 L15
  constraint parallel L13 L14
  constraint horizontal L15
  constraint parallel L16 L18
  constraint perpendicular L18 L19
  constraint perpendicular L20 L23
  constraint parallel L21 L23
  constraint parallel L20 L22
  constraint horizontal L23
  measures "d1" distance of L1.end L2.end
  measures "d2" distance of L0.end L1.end
  measures "d3" distance of L6.end L7.end
  measures "d4" distance of L13.start L12.start
  measures "d6" distance of L16.start L16.end
  measures "d7" distance of L20.start L20.end
extrude "Extrude1" add sketch "Sketch1" along normal blind 10 and the other way blind 0
ref_plane "WorkPlane1" through (0, 0, 10) normal (0, 0, 1) x (1, 0, 0)
sketch "Sketch2" plane through (0, 0, 10) normal (0, 0, 1) x (1, 0, 0)
  line L0 (62.5, -41.5) -> (-62.5, -41.5)
  line L1 (-62.5, -41.5) -> (-62.5, 41.5)
  line L2 (-62.5, 41.5) -> (62.5, 41.5)
  line L3 (62.5, 41.5) -> (62.5, -41.5)
  line L4 (62.5, -41.5) -> (-62.5, 41.5) construction
  line L5 (-62.5, -41.5) -> (62.5, 41.5) construction
  line L6 (-62.5, -41.5) -> (-62.5, 34.9)
  line L7 (62.5, 41.5) -> (-55.8, 41.5)
  line L8 (-62.5, 34.9) -> (-55.8, 41.5)
  dimension "d13" = 125
  dimension "d14" = 83
  dimension "d15" = 76.4
  dimension "d16" = 118.3
  constraint perpendicular L0 L1
  constraint parallel L0 L2
  constraint parallel L1 L3
  constraint horizontal L0
  constraint coincident L4 origin
  constraint coincident L5 origin
  constraint perpendicular L0 L6
  constraint perpendicular L3 L7
  measures "d13" distance of L1.end L2.end
  measures "d14" distance of L0.end L1.end
  measures "d15" distance of L0.end L6.end
  measures "d16" distance of L2.end L7.end
extrude "Extrude2" cut sketch "Sketch2" against normal blind 8 contours L0 L1 L2 L3 L6 L7 L8
ref_plane "WorkPlane2" through (0, 0, 10) normal (0, 0, 1) x (1, 0, 0)
sketch "Sketch3" plane through (0, 0, 10) normal (0, 0, 1) x (1, 0, 0)
  circle A0 centre (-53.3802, 52.2353) radius 3.25
  circle A1 centre (53.38, 52.2349) radius 3.25
  circle A2 centre (53.3799, -52.2347) radius 3.25
  circle A3 centre (-53.3802, -52.2349) radius 3.25
  dimension "d20" = 6.5
  dimension "d21" = 6.5
  dimension "d22" = 6.5
  dimension "d23" = 6.5
  measures "d20" diameter of A0
  measures "d21" diameter of A1
  measures "d22" diameter of A2
  measures "d23" diameter of A3
extrude "Extrude3" cut sketch "Sketch3" against normal blind 10
fillet "Fillet1" radius 5 4 edges at (68.38, -47.235, 5) (68.38, 47.235, 5) (-68.38, -47.235, 5) (-68.38, 47.235, 5)
fillet "Fillet2" radius 2 16 edges at (58.38, -47.235, 5) (58.38, -57.235, 5) (48.38, -57.235, 5) (58.38, 57.235, 5) (-48.38, -47.235, 5) (-48.38, -57.235, 5) (-58.38, -57.235, 5) (-48.38, 57.235, 5) (58.38, 47.235, 5) (-48.38, 47.235, 5) (-58.38, 57.235, 5) (48.38, 57.235, 5) (48.38, 47.235, 5) (-58.38, 47.235, 5) (48.38, -47.235, 5) (-58.38, -47.235, 5)
extrude "Extrude4" add 1 faces at (-18.6, -13.8333, 2) along direction (0, 0, 1) blind 8
ref_plane "WorkPlane3" through (0, 0, 10) normal (0, 0, 1) x (1, 0, 0)
sketch "Sketch4" plane through (0, 0, 10) normal (0, 0, 1) x (1, 0, 0)
  line L0 (63, -42) -> (-63, -42)
  line L1 (-63, -42) -> (-63, 42)
  line L2 (-63, 42) -> (63, 42)
  line L3 (63, 42) -> (63, -42)
  line L4 (63, -42) -> (-63, 42) construction
  line L5 (-63, -42) -> (63, 42) construction
  line L6 (63, -42) -> (63, 34.4)
  line L7 (-63, 42) -> (55.3, 42)
  line L8 (55.3, 42) -> (63, 34.4)
  dimension "d31" = 126
  dimension "d32" = 84
  dimension "d33" = 76.4
  dimension "d34" = 118.3
  constraint perpendicular L0 L1
  constraint parallel L0 L2
  constraint parallel L1 L3
  constraint horizontal L0
  constraint coincident L4 origin
  constraint coincident L5 origin
  constraint perpendicular L0 L6
  constraint perpendicular L1 L7
  measures "d31" distance of L1.end L2.end
  measures "d32" distance of L0.end L1.end
  measures "d33" distance of L0.start L6.end
  measures "d34" distance of L1.end L7.end
extrude "Extrude6" cut sketch "Sketch4" against normal blind 8 contours L0 L1 L2 L3 L6 L7 L8
extrude "Extrude5" cut sketch "Sketch4" against normal blind 8 contours L0 L1 L2 L3 L6 L7 L8
